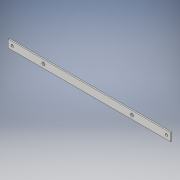
# Autodesk Inventor part: screen support
Saved by Autodesk Inventor 2018 (Build 220112000, 112)
## iProperties
Created: 2019-09-14
Part Number: screen support
Material: Generic
Document SubType Name: Modeling
Designer: Jacob
Density: 1 g/cm^3
Appearance: Default
Author: Jacob
Autodesk Inventor part; units mm, degrees
ref_plane "YZ Plane" through (0, 0, 0) normal (1, 0, 0) x (0, 1, 0)
ref_plane "XZ Plane" through (0, 0, 0) normal (0, 1, 0) x (-1, 0, 0)
ref_plane "XY Plane" through (0, 0, 0) normal (0, 0, 1) x (1, 0, 0)
sketch "Sketch1" plane through (0, 0, 0) normal (0, 0, 1) x (1, 0, 0)
  line L0 (-62.8523, 3) -> (62.8523, 3)
  line L1 (62.8523, 3) -> (62.8523, -3)
  line L2 (62.8523, -3) -> (-62.8523, -3)
  line L3 (-62.8523, -3) -> (-62.8523, 3)
  line L4 (-62.8523, 3) -> (62.8523, -3) construction
  line L5 (62.8523, 3) -> (-62.8523, -3) construction
  point P0 (0, 0)
  dimension "d0" = 6
  dimension "d1" = 125.7046
  constraints: 12 end point, 2 midpoint, 2 parallel, 1 horizontal, 1 perpendicular
  measures "d0" distance between parallel lines of L2 L0
  measures "d1" distance of L0.start L0.end
extrude "Extrusion1" add sketch "Sketch1" along normal blind 1
sketch "Sketch2" plane through (0, 0, 1) normal (0, 0, 1) x (1, 0, 0)
  line L0 (62.8523, 3) -> (-62.8523, 3) projected
  line L1 (33.0023, 3) -> (33.0023, -3) construction
  line L2 (-62.8523, -3) -> (62.8523, -3) projected
  line L3 (62.8523, -3) -> (62.8523, 3) projected
  line L4 (-35.5023, 3) -> (-35.5023, -3) construction
  line L5 (-62.8523, 3) -> (-62.8523, -3) projected
  line L6 (-62.8523, 0) -> (62.8523, 0) construction
  circle A0 centre (-35.5023, 0) radius 1.25
  circle A1 centre (33.0023, 0) radius 1.25
  line L7 (56.5023, 3) -> (56.5023, -3) construction
  line L8 (-56.5023, 3) -> (-56.5023, -3) construction
  line L9 (-59.6773, 3) -> (-59.6773, -3) construction
  line L10 (59.6773, 3) -> (59.6773, -3) construction
  circle A2 centre (59.6773, 0) radius 1
  circle A3 centre (-59.6773, 0) radius 1
  point P0 (0, 0)
  dimension "d4" = 29.85
  dimension "d5" = 27.35
  dimension "d6" = 2.5
  dimension "d7" = 2.5
  dimension "d8" = 6.35
  dimension "d9" = 6.35
  dimension "d10" = 3.175
  dimension "d11" = 3.175
  dimension "d12" = 2
  dimension "d13" = 2
  constraints: 14 end point, 14 point on line, 6 midpoint, 5 perpendicular, 4 centre point, 1 vertical
  measures "d4" distance between parallel lines of L3 L1
  measures "d5" distance between parallel lines of L4 L5
  measures "d6" diameter of A0
  measures "d7" diameter of A1
  measures "d8" distance between parallel lines of L3 L7
  measures "d9" distance between parallel lines of L5 L8
  measures "d10" distance between parallel lines of L5 L9
  measures "d11" distance between parallel lines of L3 L10
  measures "d12" diameter of A2
  measures "d13" diameter of A3
extrude "Extrusion2" cut sketch "Sketch2" against normal blind 25.4 contours A0 | A1 | A2 | A3
body "Solid1"
